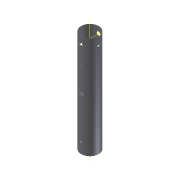
# Autodesk Inventor part: Inner shield 2
Saved by Autodesk Inventor 2015 (Build 190159000, 159)
## iProperties
Created: 2007-06-06
Part Number: Inner shield 2
Document SubType Name: Modeling
Designer: Mike
Material: Generic
Density: 1 g/cm^3
Appearance: Default
Author: Mike
Autodesk Inventor part; units mm, degrees
sketch "Sketch1" plane through (0, 0, 0) normal (0, 0, 1) x (1, 0, 0)
  circle A0 centre (0, 0) radius 85.5
  circle A1 centre (0, 0) radius 84.5
  dimension "d0" = 171
  dimension "d1" = 169
  constraints: 2 centre point, 1 coincident, 1 other
  measures "d0" diameter of A0
  measures "d1" diameter of A1
extrude "Extrusion1" add sketch "Sketch1" along normal blind 985
ref_plane "Work Plane1" through (0, 85.5, 0) normal (0, 1, 0) x (-1, 0, 0)
sketch "Sketch2" plane through (0, 85.5, 0) normal (0, 1, 0) x (-1, 0, 0)
  line L0 (-85.5, 985) -> (85.5, 985) projected
  line L1 (-85.5, 0) -> (85.5, 0) projected
  line L2 (0, 0) -> (0, 985) construction
  point P0 (0, 921.5)
  point P1 (0, 813.5)
  point P2 (0, 734)
  point P3 (0, 100)
  dimension "d4" = 100
  dimension "d5" = 63.5
  dimension "d6" = 108
  dimension "d7" = 79.5
  constraints: 4 point on line, 2 end point, 2 midpoint
  measures "d4" vertical distance of point (0, 100) L1.end
  measures "d5" vertical distance of point (0, 921.5) L0.end
  measures "d6" distance of point (0, 813.5) point (0, 921.5)
  measures "d7" distance of point (0, 734) point (0, 813.5)
hole "Hole1" at (0, 85.5, 921.5) at (0, 85.5, 813.5) at (0, 85.5, 734) at (0, 85.5, 100) direction (0, -1, 0) diameter 20 end through all
sketch "Sketch3" plane through (0, 0, 0) normal (0, 1, 0) x (-1, 0, 0)
  spline S0 degree 3 poles (0, 724) (-1.2569, 724) (-2.5967, 724.2514) (-5.0602, 725.2723) (-6.1839, 726.0417) (-7.9583, 727.8161) (-8.7277, 728.9398) (-9.7486, 731.4033) (-10, 732.7431) (-10, 735.2569) (-9.7486, 736.5967) (-8.7277, 739.0602) (-7.9583, 740.1839) (-6.1839, 741.9583) (-5.0602, 742.7277) (-2.5967, 743.7486) (-1.2569, 744) (0, 744) knots 1.508229 1.508229 1.508229 1.508229 1.885286 1.885286 2.262342 2.262342 2.6394 2.6394 3.016459 3.016459 3.393517 3.393517 3.770576 3.770576 4.147632 4.147632 4.524688 4.524688 4.524688 4.524688
  spline S1 degree 3 poles (0, 744) (1.2569, 744) (2.5967, 743.7486) (5.0602, 742.7277) (6.1839, 741.9583) (7.9583, 740.1839) (8.7277, 739.0602) (9.7486, 736.5967) (10, 735.2569) (10, 734) (10, 732.7431) (9.7486, 731.4033) (8.7277, 728.9398) (7.9583, 727.8161) (6.1839, 726.0417) (5.0602, 725.2723) (2.5967, 724.2514) (1.2569, 724) (0, 724) knots 4.524688 4.524688 4.524688 4.524688 4.901745 4.901745 5.278801 5.278801 5.655859 5.655859 6.032918 6.032918 6.032918 6.409976 6.409976 6.787035 6.787035 7.164091 7.164091 7.541147 7.541147 7.541147 7.541147
  spline S2 degree 3 poles (10, 734) (10, 734.9426) (9.7235, 736.9235) (8.5563, 739.3745) (7.5147, 740.6274) (6.6275, 741.5147) (5.625, 742.3474) (3.8544, 743.3005) (1.9279, 743.8795) (0.6285, 744) (-0.6285, 744) (-2.2532, 743.8501) (-4.8121, 742.9409) (-6.4056, 741.7365) (-7.7365, 740.4056) (-8.9407, 738.8118) (-9.8501, 736.2531) (-10, 734.6285) (-10, 733.3715) (-9.8796, 732.0722) (-9.3004, 730.1455) (-8.3475, 728.3751) (-7.5147, 727.3726) (-6.6275, 726.4853) (-5.3745, 725.4436) (-2.9233, 724.2762) (-0.9427, 724) (0.9427, 724) (2.9235, 724.2765) (5.3745, 725.4437) (6.6275, 726.4853) (7.5147, 727.3726) (8.3474, 728.375) (9.3005, 730.1457) (9.8795, 732.0721) (10, 733.3716) (10, 734) knots 0 0 0 0 0.282793 0.565586 0.754115 0.754115 0.942643 1.131172 1.319701 1.508229 1.508229 1.696758 1.979551 2.262344 2.262344 2.545137 2.82793 3.016459 3.016459 3.204988 3.393516 3.582045 3.770574 3.770574 3.959102 4.241895 4.524688 4.524688 4.807481 5.090274 5.278803 5.278803 5.467332 5.65586 5.844389 6.032918 6.032918 6.032918 6.032918
  spline S3 degree 3 poles (0, 911.5) (-1.2569, 911.5) (-2.5967, 911.7514) (-5.0602, 912.7723) (-6.1839, 913.5417) (-7.9583, 915.3161) (-8.7277, 916.4398) (-9.7486, 918.9033) (-10, 920.2431) (-10, 922.7569) (-9.7486, 924.0967) (-8.7277, 926.5602) (-7.9583, 927.6839) (-6.1839, 929.4583) (-5.0602, 930.2277) (-2.5967, 931.2486) (-1.2569, 931.5) (0, 931.5) knots 1.508229 1.508229 1.508229 1.508229 1.885286 1.885286 2.262342 2.262342 2.6394 2.6394 3.016459 3.016459 3.393517 3.393517 3.770576 3.770576 4.147632 4.147632 4.524688 4.524688 4.524688 4.524688
  spline S4 degree 3 poles (0, 931.5) (1.2569, 931.5) (2.5967, 931.2486) (5.0602, 930.2277) (6.1839, 929.4583) (7.9583, 927.6839) (8.7277, 926.5602) (9.7486, 924.0967) (10, 922.7569) (10, 921.5) (10, 920.2431) (9.7486, 918.9033) (8.7277, 916.4398) (7.9583, 915.3161) (6.1839, 913.5417) (5.0602, 912.7723) (2.5967, 911.7514) (1.2569, 911.5) (0, 911.5) knots 4.524688 4.524688 4.524688 4.524688 4.901745 4.901745 5.278801 5.278801 5.655859 5.655859 6.032918 6.032918 6.032918 6.409976 6.409976 6.787035 6.787035 7.164091 7.164091 7.541147 7.541147 7.541147 7.541147
  spline S5 degree 3 poles (10, 921.5) (10, 922.4426) (9.7235, 924.4235) (8.5563, 926.8745) (7.5147, 928.1274) (6.6275, 929.0147) (5.625, 929.8474) (3.8544, 930.8005) (1.9279, 931.3795) (0.6285, 931.5) (-0.6285, 931.5) (-2.2532, 931.3501) (-4.8121, 930.4409) (-6.4056, 929.2365) (-7.7365, 927.9056) (-8.9407, 926.3118) (-9.8501, 923.7531) (-10, 922.1285) (-10, 920.8715) (-9.8796, 919.5722) (-9.3004, 917.6455) (-8.3475, 915.8751) (-7.5147, 914.8726) (-6.6275, 913.9853) (-5.3745, 912.9436) (-2.9233, 911.7762) (-0.9427, 911.5) (0.9427, 911.5) (2.9235, 911.7765) (5.3745, 912.9437) (6.6275, 913.9853) (7.5147, 914.8726) (8.3474, 915.875) (9.3005, 917.6457) (9.8795, 919.5721) (10, 920.8716) (10, 921.5) knots 0 0 0 0 0.282793 0.565586 0.754115 0.754115 0.942643 1.131172 1.319701 1.508229 1.508229 1.696758 1.979551 2.262344 2.262344 2.545137 2.82793 3.016459 3.016459 3.204988 3.393516 3.582045 3.770574 3.770574 3.959102 4.241895 4.524688 4.524688 4.807481 5.090274 5.278803 5.278803 5.467332 5.65586 5.844389 6.032918 6.032918 6.032918 6.032918
  spline S6 degree 3 poles (0, 803.5) (-1.2569, 803.5) (-2.5967, 803.7514) (-5.0602, 804.7723) (-6.1839, 805.5417) (-7.9583, 807.3161) (-8.7277, 808.4398) (-9.7486, 810.9033) (-10, 812.2431) (-10, 814.7569) (-9.7486, 816.0967) (-8.7277, 818.5602) (-7.9583, 819.6839) (-6.1839, 821.4583) (-5.0602, 822.2277) (-2.5967, 823.2486) (-1.2569, 823.5) (0, 823.5) knots 1.508229 1.508229 1.508229 1.508229 1.885286 1.885286 2.262342 2.262342 2.6394 2.6394 3.016459 3.016459 3.393517 3.393517 3.770576 3.770576 4.147632 4.147632 4.524688 4.524688 4.524688 4.524688
  spline S7 degree 3 poles (0, 823.5) (1.2569, 823.5) (2.5967, 823.2486) (5.0602, 822.2277) (6.1839, 821.4583) (7.9583, 819.6839) (8.7277, 818.5602) (9.7486, 816.0967) (10, 814.7569) (10, 813.5) (10, 812.2431) (9.7486, 810.9033) (8.7277, 808.4398) (7.9583, 807.3161) (6.1839, 805.5417) (5.0602, 804.7723) (2.5967, 803.7514) (1.2569, 803.5) (0, 803.5) knots 4.524688 4.524688 4.524688 4.524688 4.901745 4.901745 5.278801 5.278801 5.655859 5.655859 6.032918 6.032918 6.032918 6.409976 6.409976 6.787035 6.787035 7.164091 7.164091 7.541147 7.541147 7.541147 7.541147
  spline S8 degree 3 poles (10, 813.5) (10, 814.4426) (9.7235, 816.4235) (8.5563, 818.8745) (7.5147, 820.1274) (6.6275, 821.0147) (5.625, 821.8474) (3.8544, 822.8005) (1.9279, 823.3795) (0.6285, 823.5) (-0.6285, 823.5) (-2.2532, 823.3501) (-4.8121, 822.4409) (-6.4056, 821.2365) (-7.7365, 819.9056) (-8.9407, 818.3118) (-9.8501, 815.7531) (-10, 814.1285) (-10, 812.8715) (-9.8796, 811.5722) (-9.3004, 809.6455) (-8.3475, 807.8751) (-7.5147, 806.8726) (-6.6275, 805.9853) (-5.3745, 804.9436) (-2.9233, 803.7762) (-0.9427, 803.5) (0.9427, 803.5) (2.9235, 803.7765) (5.3745, 804.9437) (6.6275, 805.9853) (7.5147, 806.8726) (8.3474, 807.875) (9.3005, 809.6457) (9.8795, 811.5721) (10, 812.8716) (10, 813.5) knots 0 0 0 0 0.282793 0.565586 0.754115 0.754115 0.942643 1.131172 1.319701 1.508229 1.508229 1.696758 1.979551 2.262344 2.262344 2.545137 2.82793 3.016459 3.016459 3.204988 3.393516 3.582045 3.770574 3.770574 3.959102 4.241895 4.524688 4.524688 4.807481 5.090274 5.278803 5.278803 5.467332 5.65586 5.844389 6.032918 6.032918 6.032918 6.032918
  spline S9 degree 3 poles (0, 90) (-1.2569, 90) (-2.5967, 90.2514) (-5.0602, 91.2723) (-6.1839, 92.0417) (-7.9583, 93.8161) (-8.7277, 94.9398) (-9.7486, 97.4033) (-10, 98.7431) (-10, 101.2569) (-9.7486, 102.5967) (-8.7277, 105.0602) (-7.9583, 106.1839) (-6.1839, 107.9583) (-5.0602, 108.7277) (-2.5967, 109.7486) (-1.2569, 110) (0, 110) knots 1.508229 1.508229 1.508229 1.508229 1.885286 1.885286 2.262342 2.262342 2.6394 2.6394 3.016459 3.016459 3.393517 3.393517 3.770576 3.770576 4.147632 4.147632 4.524688 4.524688 4.524688 4.524688
  spline S10 degree 3 poles (0, 110) (1.2569, 110) (2.5967, 109.7486) (5.0602, 108.7277) (6.1839, 107.9583) (7.9583, 106.1839) (8.7277, 105.0602) (9.7486, 102.5967) (10, 101.2569) (10, 100) (10, 98.7431) (9.7486, 97.4033) (8.7277, 94.9398) (7.9583, 93.8161) (6.1839, 92.0417) (5.0602, 91.2723) (2.5967, 90.2514) (1.2569, 90) (0, 90) knots 4.524688 4.524688 4.524688 4.524688 4.901745 4.901745 5.278801 5.278801 5.655859 5.655859 6.032918 6.032918 6.032918 6.409976 6.409976 6.787035 6.787035 7.164091 7.164091 7.541147 7.541147 7.541147 7.541147
  spline S11 degree 3 poles (10, 100) (10, 100.9426) (9.7235, 102.9235) (8.5563, 105.3745) (7.5147, 106.6274) (6.6275, 107.5147) (5.625, 108.3474) (3.8544, 109.3005) (1.9279, 109.8795) (0.6285, 110) (-0.6285, 110) (-2.2532, 109.8501) (-4.8121, 108.9409) (-6.4056, 107.7365) (-7.7365, 106.4056) (-8.9407, 104.8118) (-9.8501, 102.2531) (-10, 100.6285) (-10, 99.3715) (-9.8796, 98.0722) (-9.3004, 96.1455) (-8.3475, 94.3751) (-7.5147, 93.3726) (-6.6275, 92.4853) (-5.3745, 91.4436) (-2.9233, 90.2762) (-0.9427, 90) (0.9427, 90) (2.9235, 90.2765) (5.3745, 91.4437) (6.6275, 92.4853) (7.5147, 93.3726) (8.3474, 94.375) (9.3005, 96.1457) (9.8795, 98.0721) (10, 99.3716) (10, 100) knots 0 0 0 0 0.282793 0.565586 0.754115 0.754115 0.942643 1.131172 1.319701 1.508229 1.508229 1.696758 1.979551 2.262344 2.262344 2.545137 2.82793 3.016459 3.016459 3.204988 3.393516 3.582045 3.770574 3.770574 3.959102 4.241895 4.524688 4.524688 4.807481 5.090274 5.278803 5.278803 5.467332 5.65586 5.844389 6.032918 6.032918 6.032918 6.032918
  line L0 (-85.5, 985) -> (85.5, 985)
  line L1 (-85.5, 0) -> (85.5, 0)
  line L2 (0, 0) -> (0, 674.1527) construction
  line L3 (-10, 519) -> (10, 519)
  line L4 (25, 504) -> (25, 504)
  line L5 (10, 489) -> (-10, 489)
  line L6 (-25, 504) -> (-25, 504)
  arc A0 (10, 489) -> (25, 504) centre (10, 504) ccw
  arc A1 (-25, 504) -> (-10, 489) centre (-10, 504) ccw
  arc A2 (-10, 519) -> (-25, 504) centre (-10, 504) ccw
  arc A3 (25, 504) -> (10, 519) centre (10, 504) ccw
  point P0 (-25, 519)
  point P1 (25, 519)
  point P2 (-25, 489)
  dimension "d15" = 30
  dimension "d16" = 50
  dimension "d19" = 15
  dimension "d20" = 481
  constraints: 14 end point, 8 point on circle, 8 tangent, 6 point on line, 4 centre point, 3 equal radius, 2 parallel, 2 perpendicular, 1 horizontal, 1 midpoint, 21 other
  measures "d15" distance of point (-25, 489) point (-25, 519)
  measures "d16" distance of point (-25, 519) point (25, 519)
  measures "d19" radius of A0
  measures "d20" vertical distance of L0.end A0.centre
extrude "Extrusion2" cut sketch "Sketch3" against normal blind 100 contours L3 A3 A0 L5 A1 A2
ref_plane "Work Plane2" through (85.5, 0, 0) normal (1, 0, 0) x (0, 1, 0)
sketch "Sketch4" plane through (85.5, 0, 0) normal (1, 0, 0) x (0, 1, 0)
  line L0 (-85.5, 985) -> (85.5, 985) projected
  line L1 (0, 985) -> (0, 666.0394) construction
  point P0 (0, 921.5)
  dimension "d23" = 63.5
  constraints: 2 end point, 1 midpoint, 1 perpendicular, 1 point on line
  measures "d23" vertical distance of point (0, 921.5) L0.end
hole "Hole2" at (85.5, 0, 921.5) direction (-1, 0, 0) diameter 45 depth 8 tip angle 118
ref_plane "Work Plane3" through (-85.5, 0, 0) normal (1, 0, 0) x (0, 1, 0)
sketch "Sketch5" plane through (-85.5, 0, 0) normal (1, 0, 0) x (0, 1, 0)
  line L0 (-85.5, 985) -> (85.5, 985) projected
  line L1 (0, 985) -> (0, 697.9366)
  line L2 (0, 813.5) -> (59.5417, 813.5) construction
  point P0 (20, 813.5)
  point P1 (0, 833.5)
  point P2 (-20, 813.5)
  point P3 (0, 793.5)
  dimension "d31" = 171.5
  dimension "d32" = 20
  dimension "d35" = 360
  constraints: 4 end point, 2 perpendicular, 2 point on line, 1 midpoint, 5 other
  measures "d31" distance of L2.start L1.start
  measures "d32" distance of point (20, 813.5) L2.start
hole "Hole3" at (-85.5, 20, 813.5) at (-85.5, 0, 833.5) at (-85.5, -20, 813.5) at (-85.5, 0, 793.5) direction (1, 0, 0) diameter 20 depth 10 tip angle 118
sketch "Sketch6" plane through (0, 85.5, 0) normal (0, 1, 0) x (-1, 0, 0)
  circle A0 centre (0, 921.5) radius 10
  line L0 (-85.5, 985) -> (85.5, 985) projected
  point P0 (0, 0)
  dimension "d44" = 20
  dimension "d45" = 63.5
  constraints: 1 centre point
  measures "d44" diameter of A0
  measures "d45" distance from line of L0 A0.centre
sketch "Sketch7" plane through (0, 85.5, 0) normal (0, 1, 0) x (-1, 0, 0)
  circle A0 centre (0, 921.5) radius 17.5
  line L0 (-85.5, 985) -> (85.5, 985) projected
  point P0 (0, 0)
  dimension "d46" = 35
  dimension "d47" = 63.5
  constraints: 1 centre point
  measures "d46" diameter of A0
  measures "d47" distance from line of A0.centre L0
extrude "Extrusion4" cut sketch "Sketch7" against normal through all
body "Solid1"
